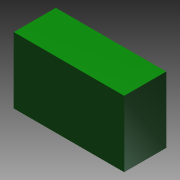
# Autodesk Inventor part: UB16NKG015F-NR
Saved by Autodesk Inventor 2015 SP1 (Build 190203100, 203)
## iProperties
Category: Electrical
Company: Autodesk Inc.
Created: 2014-12-16
Part Number: UB16NKG015F-NR
Catalog Web Link: http://www.nkkswitches.com/
Description: UB_ill_spot-Illuminated Pushbuttons - Series UB
Vendor: NKK Switches
Document SubType Name: Modeling
Designer: Autodesk Inc.
Manufacturer: NKKSWITCHES
Mass: 0.02857 g
Surface Area: 0.604786 cm^2
Volume: 0.02857 cm^3
Density: 1 g/cm^3
Material: Generic
Appearance: PSOLRGB-0-255-0
PSOL_IDENT_2: LINEID=10},{LINESUBID=-1},{WBVAR=L}  {NB=UB5F-spot},{LINA=UB5F-spot},{KT=DUMMY},{SRS=UB},{L=5F},{COL=
PSOL_IDENT_3: 0.00,1.00,0.00,0.00},{PN=UB5F}
SUPPLIER: NKKSWITCHES
Title: UB5F-spot
Author: Autodesk Inc.
Comments: Illuminated Pushbuttons - Series UB
Autodesk Inventor part; units mm, degrees
sketch "Sketch_1" plane through (0, 0, 0) normal (0, 1, 0) x (-1, 0, 0)
  line L0 (2.5019, -0.9525) -> (2.5019, 0.9525)
  line L1 (2.5019, 0.9525) -> (-2.5019, 0.9525)
  line L2 (-2.5019, 0.9525) -> (-2.5019, -0.9525)
  line L3 (-2.5019, -0.9525) -> (2.5019, -0.9525)
  constraints: 8 end point
extrude "Extrusion1" add sketch "Sketch_1" along normal blind 2.9972
ref_plane "CAP_XY" through (0, 0, 0) normal (0, 1, 0) x (1, 0, 0)
ref_plane "CAP_YZ" through (0, 0, 0) normal (1, 0, 0) x (0, 0, -1)
ref_plane "CAP_ZX" through (0, 0, 0) normal (0, 0, -1) x (0, 1, 0)
body "Solid1"
